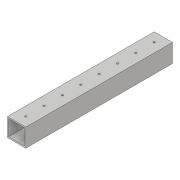
# Autodesk Inventor part: Drive Rail 1 upright 2
Saved by Autodesk Inventor 2018 (Build 220112000, 112)
## iProperties
Created: 2017-12-18
Part Number: Drive Rail 1 upright 2
Material: Generic
Document SubType Name: Modeling
Designer: dsayers
Density: 1 g/cm^3
Appearance: Default
Author: dsayers
Autodesk Inventor part; units mm, degrees
ref_plane "YZ Plane" through (0, 0, 0) normal (1, 0, 0) x (0, 1, 0)
ref_plane "XZ Plane" through (0, 0, 0) normal (0, 1, 0) x (-1, 0, 0)
ref_plane "XY Plane" through (0, 0, 0) normal (0, 0, 1) x (1, 0, 0)
sketch "Sketch1" plane through (0, 0, 0) normal (0, 0, 1) x (1, 0, 0)
  line L0 (0, 0) -> (25.4, 0)
  line L1 (25.4, 0) -> (25.4, 25.4)
  line L2 (25.4, 25.4) -> (0, 25.4)
  line L3 (0, 25.4) -> (0, 0)
  line L4 (1.5875, 23.8125) -> (23.6267, 23.8125)
  line L5 (23.6267, 23.8125) -> (23.6267, 2.0041)
  line L6 (23.6267, 2.0041) -> (1.5875, 2.0041)
  line L7 (1.5875, 2.0041) -> (1.5875, 23.8125)
  dimension "d0" = 25.4
  dimension "d1" = 25.4
  dimension "d2" = 1.5875
  dimension "d3" = 1.5875
  constraints: 16 end point, 4 parallel, 2 horizontal, 2 perpendicular
  measures "d0" distance of L1.end L2.end
  measures "d1" distance of L2.end L0.start
  measures "d2" distance between parallel lines of L2 L4
  measures "d3" distance between parallel lines of L3 L7
extrude "Extrusion1" add sketch "Sketch1" along normal blind 203.2
sketch "Sketch2" plane through (0, 25.4, 0) normal (0, 1, 0) x (1, 0, 0)
  line L0 (25.4, 0) -> (0, 0) projected
  line L1 (25.4, 0) -> (25.4, -203.2) projected
  point P0 (12.7, -12.7)
  point P1 (12.7, -38.1)
  point P2 (12.7, -63.5)
  point P3 (12.7, -88.9)
  point P4 (12.7, -114.3)
  point P5 (12.7, -139.7)
  point P6 (12.7, -165.1)
  point P7 (12.7, -190.5)
  point P8 (12.7, -215.9)
  point P9 (12.7, -241.3)
  point P10 (12.7, -266.7)
  point P11 (12.7, -292.1)
  point P12 (12.7, -317.5)
  point P13 (12.7, -342.9)
  point P14 (12.7, -368.3)
  dimension "d6" = 12.7
  dimension "d7" = 12.7
  dimension "d10" = 25.4
  constraints: 1 vertical, 14 other
  measures "d6" distance from line of L0 point (12.7, -12.7)
  measures "d7" distance from line of L1 point (12.7, -12.7)
  measures "d10" distance of point (12.7, -12.7) point (12.7, -38.1)
hole "Hole1" at (12.7, 25.4, 12.7) at (12.7, 25.4, 38.1) at (12.7, 25.4, 63.5) at (12.7, 25.4, 88.9) at (12.7, 25.4, 114.3) at (12.7, 25.4, 139.7) at (12.7, 25.4, 165.1) at (12.7, 25.4, 190.5) at (12.7, 25.4, 215.9) at (12.7, 25.4, 241.3) at (12.7, 25.4, 266.7) at (12.7, 25.4, 292.1) at (12.7, 25.4, 317.5) at (12.7, 25.4, 342.9) at (12.7, 25.4, 368.3) direction (0, -1, 0) diameter 2.54 depth 25.4 tip angle 118
body "Solid1"
